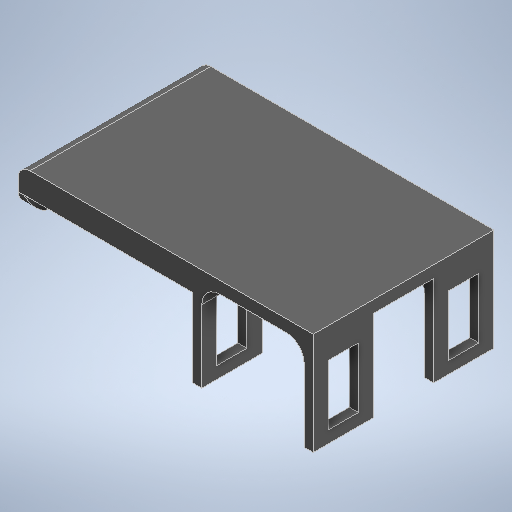
# Autodesk Inventor part: connetcor_female_cover
Saved by Autodesk Inventor 2026.1 (Build 301233020, 233B)
## iProperties
Created: 2025-09-28
Part Number: connetcor_female_cover
Material: 一般
Document SubType Name: Modeling
Designer: hibik
Density: 1 g/cm^3
Appearance: 既定
Author: hibik
Autodesk Inventor part; units mm, degrees
ref_plane "YZ Plane" through (0, 0, 0) normal (1, 0, 0) x (0, 1, 0)
ref_plane "XZ Plane" through (0, 0, 0) normal (0, 1, 0) x (-1, 0, 0)
ref_plane "XY Plane" through (0, 0, 0) normal (0, 0, 1) x (1, 0, 0)
sketch "スケッチ1" plane through (0, 0, 0) normal (0, 0, 1) x (1, 0, 0)
  line L0 (-10, 17) -> (0, 17)
  line L1 (0, 17) -> (0, 15)
  line L2 (0, 15) -> (-10, 15)
  line L3 (-10, 15) -> (-10, 17)
  line L4 (0, -3.4) -> (0, 20.4) projected
  point P0 (0, 0)
  dimension "d0" = 10
  dimension "d1" = 2
  dimension "d2" = 15
  constraints: 8 end point, 2 parallel, 1 collinear, 1 horizontal, 1 perpendicular
  measures "d0" distance of L0.start L0.end
  measures "d1" distance of L2.end L0.start
  measures "d2" distance from line of point (0, 0) L2
extrude "押し出し1" add sketch "スケッチ1" along normal blind 5
sketch "スケッチ2" plane through (0, 0, 5) normal (0, 0, 1) x (1, 0, 0)
  line L0 (0, 17) -> (-10, 17) projected
  line L1 (-10, 17) -> (-8.5, 17)
  line L2 (-8.5, 17) -> (-8.5, 0)
  line L3 (-8.5, 0) -> (-10, 0)
  line L4 (-10, 0) -> (-10, 17)
  line L5 (-10, 15) -> (0, 15) projected
  line L6 (0, 15) -> (0, 17) projected
  line L7 (0, 17) -> (-10, 17) projected
  line L8 (-10, 17) -> (-10, 15) projected
  point P0 (0, 0)
  point P1 (-8.5, 15)
  dimension "d5" = 1.5
  constraints: 8 end point, 2 parallel, 1 horizontal, 1 perpendicular, 1 point on line
  measures "d5" distance of L2.end L3.end
extrude "押し出し2" add sketch "スケッチ2" along normal blind 10
sketch "スケッチ3" plane through (-8.5, 0, 5) normal (1, 0, 0) x (0, 0, -1)
  line L0 (-7.5, 12) -> (-2.5, 12)
  line L1 (-2.5, 12) -> (-2.5, 2)
  line L2 (-2.5, 2) -> (-7.5, 2)
  line L3 (-7.5, 2) -> (-7.5, 12)
  line L4 (0, 0) -> (-10, 0) projected
  line L5 (0, 15) -> (-10, 15) projected
  point P0 (5, 0)
  point P1 (-5, 2)
  point P2 (-5, 0)
  dimension "d8" = 2
  dimension "d9" = 5
  dimension "d13" = 3
  constraints: 8 end point, 2 midpoint, 2 parallel, 1 horizontal, 1 perpendicular, 1 vertical alignment
  measures "d8" distance between parallel lines of L4 L2
  measures "d9" distance of L1.end L2.end
  measures "d13" distance between parallel lines of L5 L0
extrude "押し出し3" cut sketch "スケッチ3" against normal through all
fillet "フィレット1" radius 3 1 edges at (-8.5, 15, 10)
mirror "ミラー1" about plane through (0, 15, 0) normal (1, 0, 0)
mirror "ミラー2" about plane through (-5, 16, 0) normal (0, 0, -1)
sketch "スケッチ4" plane through (0, 0, 15) normal (0, 0, 1) x (1, 0, 0)
  line L0 (-10, 17) -> (-10, 0) projected
  line L1 (-10, 17) -> (-39, 17)
  line L2 (-39, 17) -> (-39, 13)
  line L3 (-39, 13) -> (-10, 13)
  line L4 (-10, 13) -> (-10, 17)
  line L5 (-39, 17) -> (-36, 17)
  line L6 (-36, 17) -> (-36, 11)
  line L7 (-36, 11) -> (-39, 11)
  line L8 (-39, 11) -> (-39, 17)
  point P0 (0, 0)
  point P1 (-36, 13)
  dimension "d14" = 4
  dimension "d15" = 3
  dimension "d16" = 26
  dimension "d17" = 6
  constraints: 16 end point, 4 parallel, 2 horizontal, 2 perpendicular
  measures "d14" distance of L1.end L2.end
  measures "d15" distance of L6.end L7.end
  measures "d16" distance between parallel lines of L0 L6
  measures "d17" distance of L7.end L1.end
extrude "押し出し4" add sketch "スケッチ4" against normal up to surface (30 mm away)
fillet "フィレット2" radius 2 1 edges at (-39, 17, 0)
fillet "フィレット3" radius 2 4 edges at (-36, 12, 15) (-37.5, 11, 15) (-37.5, 11, -15) (-36, 12, -15)
